honeycomb design_v1 (Autodesk Fusion 360 design; units mm, degrees)
Autodesk Fusion 360 part; units mm, degrees
note: some values were not read from the file. Chosen so that the rebuilt part matches the saved one: which bodies a step acts on. Set by a fixed rule: which sketch regions a step uses.
sketch "Sketch1" plane through (0, 0, 0) normal (1, 0, 0) x (0, 1, 0)
  line L0 (5.22, 16.9178) -> (-1.5257, 24.1633) construction
  line L1 (-1.7756, 17.1677) -> (5.4699, 23.9134) construction
  line L2 (6.4544, 22.3499) -> (-2.76, 18.7312) construction
  line L3 (3.6565, 15.9334) -> (0.0378, 25.1478) construction
  line L4 (-2.5283, 15.5845) -> (-6.0283, 21.6467)
  line L5 (-6.0283, 21.6467) -> (0.0339, 25.1467)
  line L6 (0.0339, 25.1467) -> (3.5339, 19.0845)
  line L7 (3.5339, 19.0845) -> (-2.5283, 15.5845)
  line L8 (-2.5283, 15.5845) -> (0.0339, 25.1467) construction
  line L9 (-6.0283, 21.6467) -> (3.5339, 19.0845) construction
  line L10 (0.9828, 21.6396) -> (-6.0172, 21.6396)
  line L11 (-6.0172, 21.6396) -> (-6.0172, 14.6396)
  line L12 (-6.0172, 14.6396) -> (0.9828, 14.6396)
  line L13 (0.9828, 14.6396) -> (0.9828, 21.6396)
  line L14 (0.9828, 21.6396) -> (-6.0172, 14.6396) construction
  line L15 (-6.0172, 21.6396) -> (0.9828, 14.6396) construction
  line L16 (3.5424, 17.1986) -> (0.0424, 11.1365)
  line L17 (0.0424, 11.1365) -> (-6.0198, 14.6365)
  line L18 (-6.0198, 14.6365) -> (-2.5198, 20.6986)
  line L19 (-2.5198, 20.6986) -> (3.5424, 17.1986)
  line L20 (3.5424, 17.1986) -> (-6.0198, 14.6365) construction
  line L21 (0.0424, 11.1365) -> (-2.5198, 20.6986) construction
  line L22 (2.601, 15.5846) -> (-3.4612, 19.0846)
  line L23 (-3.4612, 19.0846) -> (0.0388, 25.1468)
  line L24 (0.0388, 25.1468) -> (6.101, 21.6468)
  line L25 (6.101, 21.6468) -> (2.601, 15.5846)
  line L26 (2.601, 15.5846) -> (0.0388, 25.1468) construction
  line L27 (-3.4612, 19.0846) -> (6.101, 21.6468) construction
  line L28 (0, 27.3) -> (0, 26.3)
  line L29 (6.099, 14.6438) -> (-0.901, 14.6438)
  line L30 (-0.901, 14.6438) -> (-0.901, 21.6438)
  line L31 (-0.901, 21.6438) -> (6.099, 21.6438)
  line L32 (6.099, 21.6438) -> (6.099, 14.6438)
  line L33 (6.099, 14.6438) -> (-0.901, 21.6438) construction
  line L34 (-0.901, 14.6438) -> (6.099, 21.6438) construction
  line L35 (2.5961, 20.7094) -> (-3.4661, 17.2094)
  line L36 (-3.4661, 17.2094) -> (0.0339, 11.1472)
  line L37 (0.0339, 11.1472) -> (6.0961, 14.6472)
  line L38 (6.0961, 14.6472) -> (2.5961, 20.7094)
  line L39 (2.5961, 20.7094) -> (0.0339, 11.1472) construction
  line L40 (-3.4661, 17.2094) -> (6.0961, 14.6472) construction
  point P0 (1.8472, 20.5406)
  point P1 (1.8472, 20.5406)
  point P2 (-1.2472, 20.3656)
  point P3 (-2.5172, 18.1396)
  point P4 (-1.2387, 15.9176)
  point P5 (1.3199, 20.3657)
  point P6 (2.599, 18.1438)
  point P7 (1.315, 15.9283)
  constraint coincident L0 P1
  constraint coincident L1 P1
  constraint coincident L2 P1
  constraint coincident L3 P1
  constraint coincident P1 P0
  constraint perpendicular L4 L5
  constraint parallel L4 L6
  constraint parallel L5 L7
  constraint coincident L8 P2
  constraint coincident L9 P2
  constraint horizontal L10
  constraint perpendicular L10 L11
  constraint parallel L10 L12
  constraint parallel L11 L13
  constraint coincident L14 P3
  constraint coincident L15 P3
  constraint perpendicular L16 L17
  constraint parallel L16 L18
  constraint parallel L17 L19
  constraint coincident L20 P4
  constraint coincident L21 P4
  constraint perpendicular L22 L23
  constraint parallel L22 L24
  constraint parallel L23 L25
  constraint coincident L26 P5
  constraint coincident L27 P5
  constraint vertical L28
  constraint horizontal L29
  constraint perpendicular L29 L30
  constraint parallel L29 L31
  constraint parallel L30 L32
  constraint coincident L33 P6
  constraint coincident L34 P6
  constraint perpendicular L35 L36
  constraint parallel L35 L37
  constraint parallel L36 L38
  constraint coincident L39 P7
  constraint coincident L40 P7
extrude "Extrude1" add sketch "Sketch1" along normal blind 3 makes body 1
copy_body "CopyPasteBodies1" bodies 1 makes body 2
move_body "Move1" bodies 2 to x (1, 0, 0) y (0, 1, 0) z (0, 0, 1) at (0, 0, 0)
move_body "Move2" bodies 2 to x (1, 0, 0) y (0, 1, 0) z (0, 0, 1) at (0, 17, 0)
move_body "Move3" bodies 2 to x (1, 0, 0) y (0, 1, 0) z (0, 0, 1) at (0, 2.116, 0)
copy_body "CopyPasteBodies2" bodies 2 makes body 3
move_body "Move4" bodies 3 to x (1, 0, 0) y (0, 1, 0) z (0, 0, 1) at (0, 0, 0)
move_body "Move5" bodies 3 to x (1, 0, 0) y (0, 1, 0) z (0, 0, 1) at (-0.7217, -8.6394, -12.9936)
sketch "Sketch2" plane through (3, 0, 0) normal (1, 0, 0) x (0, 1, 0)
  line L0 (-6.0172, 21.6275) -> (-6.0172, 14.641)
  line L1 (-6.0172, 14.641) -> (-6.0198, 14.6365)
  line L2 (-6.0198, 14.6365) -> (0.0424, 11.1365)
  line L3 (0.0424, 11.1365) -> (0.056, 11.16)
  line L4 (0.056, 11.16) -> (6.0902, 14.6438)
  line L5 (6.0902, 14.6438) -> (6.099, 14.6438)
  line L6 (6.099, 14.6438) -> (6.099, 21.6433)
  line L7 (6.099, 21.6433) -> (6.101, 21.6468)
  line L8 (6.101, 21.6468) -> (0.0388, 25.1468)
  line L9 (0.0388, 25.1468) -> (0.0363, 25.1425)
  line L10 (0.0363, 25.1425) -> (0.0339, 25.1467)
  line L11 (0.0339, 25.1467) -> (-6.0283, 21.6467)
  line L12 (-6.0283, 21.6467) -> (-6.0172, 21.6275)
  line L13 (6.099, 18.9332) -> (9.599, 18.9332)
  line L14 (7.849, 18.9332) -> (7.849, -3.2442)
  dimension "d22" = 3.5
  constraint coincident L6 L13.start
  constraint perpendicular L6 L13
  constraint midpoint L13 L14.start
  constraint perpendicular L13 L14
  measures "d22" distance of L13.start L13.end
move_body "Move6" bodies 3 to x (1, 0, 0) y (0, 1, 0) z (0, 0, 1) at (0, -1, 0)
move_body "Move7" bodies 3 to x (1, 0, 0) y (0, 1, 0) z (0, 0, 1) at (0, 0, -2)
move_body "Move8" bodies 2 to x (1, 0, 0) y (0, 1, 0) z (0, 0, 1) at (0, -3.5, 0)
move_body "Move9" bodies 3 to x (1, 0, 0) y (0, 1, 0) z (0, 0, 1) at (0, -2, 0)
move_body "Move10" bodies 3 to x (1, 0, 0) y (0, 1, 0) z (0, 0, 1) at (0, 0.34, 0)
move_body "Move11" bodies 3 to x (1, 0, 0) y (0, 1, 0) z (0, 0, 1) at (0, 0, 1.5)
sketch "Sketch3" plane through (0, 0, 0) normal (1, 0, 0) x (0, 1, 0)
pattern_linear "R-Pattern1" count 1 spacing 0 along (0, 0.866025, -0.5) count 5 spacing 15.625 along (0, 1, 0) of bodies 1 3 makes body 4 at (0, 17.6824, 19.305) makes body 5 at (0, 33.3074, 19.305) makes body 6 at (0, 48.9324, 19.305) makes body 7 at (0, 64.5574, 19.305) makes body 8 at (-0.7217, 25.499, 5.8114) makes body 9 at (-0.7217, 41.124, 5.8114) makes body 10 at (-0.7217, 56.749, 5.8114) makes body 11 at (-0.7217, 72.374, 5.8114)
pattern_linear "R-Pattern2" count 1 spacing 0 along (1, 0, 0) count 2 spacing 27 along (0, 0, -1) of bodies 1 3 7 5 6 4 11 8 10 9 makes body 12 at (0, 2.0574, -7.695) makes body 13 at (-0.7217, 9.874, -21.1886) makes body 14 at (0, 17.6824, -7.695) makes body 15 at (0, 33.3074, -7.695) makes body 16 at (0, 48.9324, -7.695) makes body 17 at (0, 64.5574, -7.695) makes body 18 at (-0.7217, 25.499, -21.1886) makes body 19 at (-0.7217, 41.124, -21.1886) makes body 20 at (-0.7217, 56.749, -21.1886) makes body 21 at (-0.7217, 72.374, -21.1886)
sketch "Sketch4" plane through (3, 0, 0) normal (1, 0, 0) x (0, 1, 0)
  line L0 (56.4828, 21.6275) -> (56.4828, 14.641)
  line L1 (56.4828, 14.641) -> (56.4802, 14.6365)
  line L2 (56.4802, 14.6365) -> (62.5424, 11.1365)
  line L3 (62.5424, 11.1365) -> (62.556, 11.16)
  line L4 (62.556, 11.16) -> (68.5902, 14.6438)
  line L5 (68.5902, 14.6438) -> (68.599, 14.6438)
  line L6 (68.599, 14.6438) -> (68.599, 21.6433)
  line L7 (68.599, 21.6433) -> (68.601, 21.6468)
  line L8 (68.601, 21.6468) -> (62.5388, 25.1468)
  line L9 (62.5388, 25.1468) -> (62.5363, 25.1425)
  line L10 (62.5363, 25.1425) -> (62.5339, 25.1467)
  line L11 (62.5339, 25.1467) -> (56.4717, 21.6467)
  line L12 (56.4717, 21.6467) -> (56.4828, 21.6275)
